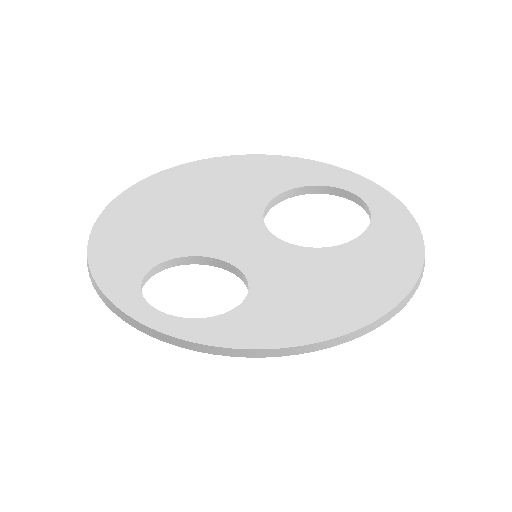
# Autodesk Inventor part: metal_base_plate
Saved by Autodesk Inventor 2025 (Build 290162000, 162)
## iProperties
Created: 2026-01-27
Part Number: metal_base_plate
Material: Generic
Document SubType Name: Modeling
Designer: MK92
Density: 1 g/cm^3
Appearance: Default
Author: MK92
Autodesk Inventor part; units mm, degrees
ref_plane "YZ Plane" through (0, 0, 0) normal (1, 0, 0) x (0, 1, 0)
ref_plane "XZ Plane" through (0, 0, 0) normal (0, 1, 0) x (-1, 0, 0)
ref_plane "XY Plane" through (0, 0, 0) normal (0, 0, 1) x (1, 0, 0)
sketch "Sketch1" plane through (0, 0, 0) normal (0, 1, 0) x (-1, 0, 0)
  point P0 (0, 0)
sketch "Sketch2" plane through (0, 0, 0) normal (0, 1, 0) x (-1, 0, 0)
  circle A0 centre (0, 0) radius 25.4
  circle A1 centre (0, 0) radius 13
  circle A2 centre (0, 13) radius 8.1
  circle A3 centre (0, -13) radius 8.1
  dimension "d0" = 50.8
  dimension "d1" = 26
  dimension "d2" = 16.2
  dimension "d3" = 16.2
  constraints: 4 centre point, 2 coincident, 2 point on circle
  measures "d0" diameter of A0
  measures "d1" diameter of A1
  measures "d2" diameter of A2
  measures "d3" diameter of A3
extrude "Extrusion1" add sketch "Sketch2" along normal blind 1.5 contours A0 | A1 A3 A2
body "Solid1"
